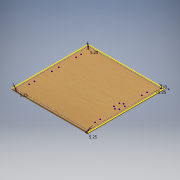
# Autodesk Inventor part: Floor
Saved by Autodesk Inventor 2019 (Build 230136000, 136)
## iProperties
Created: 2019-08-18
Part Number: Floor
Material: Generic
Document SubType Name: Modeling
Designer: Bruno
Density: 1 g/cm^3
Appearance: Default
Author: Bruno
Autodesk Inventor part; units mm, degrees
ref_plane "YZ Plane" through (0, 0, 0) normal (1, 0, 0) x (0, 1, 0)
ref_plane "XZ Plane" through (0, 0, 0) normal (0, 1, 0) x (-1, 0, 0)
ref_plane "XY Plane" through (0, 0, 0) normal (0, 0, 1) x (1, 0, 0)
sketch "Sketch1" plane through (0, 0, 0) normal (0, 1, 0) x (-1, 0, 0)
  line L0 (220, -220) -> (-220, -220)
  line L1 (-220, -220) -> (-220, 220)
  line L2 (-220, 220) -> (220, 220)
  line L3 (220, 220) -> (220, -220)
  line L4 (160, -160) -> (-160, -160)
  line L5 (-160, -160) -> (-160, 160)
  line L6 (-160, 160) -> (160, 160)
  line L7 (160, 160) -> (160, -160)
  line L8 (0, 42.2223) -> (0, -35.1237) construction
  line L9 (40.4991, 0) -> (-29.63, 0) construction
  point P0 (0, 0)
  dimension "d0" = 440
  dimension "d1" = 320
  dimension "d2" = 320
  dimension "d3" = 440
  constraints: 20 end point, 4 parallel, 3 horizontal, 2 perpendicular, 2 point on line, 1 vertical, 4 other
  measures "d0" distance of L0.start L0.end
  measures "d1" distance of L4.start L4.end
  measures "d2" distance of L6.end L4.start
  measures "d3" distance of L0.end L1.end
extrude "Extrusion1" add sketch "Sketch1" along normal blind 8 contours L0 L1 L2 L3 | L4 L5 L6 L7
sketch "Sketch3" plane through (0, 8, 0) normal (0, 1, 0) x (1, 0, 0)
  circle A0 centre (-190, -150) radius 2.5
  circle A1 centre (-190, -120) radius 2.5
  circle A2 centre (-190, -20) radius 2.125
  circle A3 centre (-190, 20) radius 2.125
  circle A4 centre (-190, 120) radius 2.5
  circle A5 centre (-190, 150) radius 2.5
  circle A6 centre (190, 120) radius 2.5
  circle A7 centre (190, 150) radius 2.5
  circle A8 centre (190, -150) radius 2.5
  circle A9 centre (190, -120) radius 2.5
  circle A10 centre (180, -25) radius 2.5
  circle A11 centre (195.5, -15.5) radius 2.5
  circle A12 centre (195.5, 15.5) radius 2.5
  circle A13 centre (180, 25) radius 2.5
  circle A14 centre (164.5, -15.5) radius 2.5
  circle A15 centre (164.5, 15.5) radius 2.5
  circle A16 centre (210, 210) radius 2.625
  circle A17 centre (210, -210) radius 2.625
  circle A18 centre (-210, -210) radius 2.625
  circle A19 centre (-210, 210) radius 2.625
  line L0 (210, 210) -> (210, -210) construction
  line L1 (210, -210) -> (-210, -210) construction
  line L2 (-210, -210) -> (-210, 210) construction
  line L3 (-210, 210) -> (210, 210) construction
  line L4 (210, 171.5822) -> (220, 171.5822)
  line L5 (220, -220) -> (220, 220) projected
  line L6 (-210, 160.3384) -> (-220, 160.3384)
  line L7 (-220, 220) -> (-220, -220) projected
  line L8 (220, 220) -> (-220, 220) projected
  line L9 (-109.669, 220) -> (-109.669, 210)
  line L10 (-109.2567, -210) -> (-109.2567, -220)
  dimension "d28" = 5.25
  dimension "d29" = 5.25
  dimension "d30" = 5.25
  dimension "d31" = 5.25
  dimension "d32" = 10
  constraints: 20 centre point, 16 end point, 7 point on line, 4 equal length, 4 perpendicular, 2 horizontal, 2 vertical, 32 other
  measures "d28" diameter of A16
  measures "d29" diameter of A17
  measures "d30" diameter of A18
  measures "d31" diameter of A19
  measures "d32" distance of L4.start L4.end
extrude "Extrusion2" cut sketch "Sketch3" against normal through all
body "Solid1"
